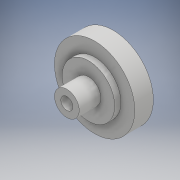
# Autodesk Inventor part: Arm - 608 bearing cap [Med]
Saved by Autodesk Inventor 2017 (Build 210142000, 142)
## iProperties
Created: 2016-08-10
Part Number: Arm - 608 bearing cap [Med]
Material: Generic
Document SubType Name: Modeling
Designer: Ali
Density: 1 g/cm^3
Appearance: Default
Author: Ali
Autodesk Inventor part; units mm, degrees
ref_plane "YZ Plane" through (0, 0, 0) normal (1, 0, 0) x (0, 1, 0)
ref_plane "XZ Plane" through (0, 0, 0) normal (0, 1, 0) x (-1, 0, 0)
ref_plane "XY Plane" through (0, 0, 0) normal (0, 0, 1) x (1, 0, 0)
sketch "Sketch1" plane through (0, 0, 0) normal (0, 1, 0) x (-1, 0, 0)
  circle A0 centre (0, 0) radius 8.5
  dimension "d0" = 17
  constraints: 1 centre point, 1 coincident
  measures "d0" diameter of A0
extrude "Extrusion1" add sketch "Sketch1" along normal blind 2
sketch "Sketch2" plane through (0, 2, 0) normal (0, 1, 0) x (1, 0, 0)
  circle A0 centre (0, 0) radius 13
  dimension "d3" = 26
  constraints: 1 centre point, 1 coincident
  measures "d3" diameter of A0
extrude "Extrusion2" add sketch "Sketch2" along normal blind 6
sketch "Sketch3" plane through (0, 0, 0) normal (0, -1, 0) x (1, 0, 0)
  circle A0 centre (0, 0) radius 4
  dimension "d6" = 8
  constraints: 1 centre point, 1 coincident
  measures "d6" diameter of A0
extrude "Extrusion3" add sketch "Sketch3" along normal blind 7
sketch "Sketch4" plane through (0, -7, 0) normal (0, -1, 0) x (1, 0, 0)
  point P0 (0, 0)
  point P1 (0, 0)
  constraints: 1 coincident
hole "Hole1" at (0, -7, 0) direction (0, 1, 0) diameter 3.9 depth 10 tip angle 118
sketch "Sketch6" plane through (0, 8, 0) normal (0, 1, 0) x (1, 0, 0)
  line L0 (5, 0) -> (-5, 0) construction
  line L1 (5, 0.9) -> (-5, 0.9)
  line L2 (-5, -0.9) -> (5, -0.9)
  arc A0 (5, -0.9) -> (5, 0.9) centre (5, 0) ccw
  arc A1 (-5, 0.9) -> (-5, -0.9) centre (-5, 0) ccw
  point P0 (0, 0)
  point P1 (0, 0)
  dimension "d24" = 1.8
  dimension "d25" = 10
  constraints: 8 end point, 4 point on circle, 4 tangent, 2 centre point, 1 coincident, 1 horizontal, 1 midpoint, 1 parallel
  measures "d24" diameter of A1
  measures "d25" distance of L0.end L0.start
extrude "Extrusion5" cut sketch "Sketch6" against normal blind 5
sketch "Sketch7" plane through (0, 8, 0) normal (0, 1, 0) x (1, 0, 0)
  line L0 (0.9699, -12.5028) -> (-0.9699, -12.5028)
  line L1 (-0.9699, -12.5028) -> (-0.9699, -13.4972)
  line L2 (-0.9699, -13.4972) -> (0.9699, -13.4972)
  line L3 (0.9699, -13.4972) -> (0.9699, -12.5028)
  circle A0 centre (0, 0) radius 13 projected
  line L4 (0.9699, -12.5028) -> (-0.9699, -13.4972) construction
  line L5 (-0.9699, -12.5028) -> (0.9699, -13.4972) construction
  circle A1 centre (0, 0) radius 13 projected
  line L6 (0, -13) -> (0, 0) construction
  constraints: 14 end point, 2 midpoint, 2 parallel, 1 horizontal, 1 perpendicular, 1 vertical, 1 vertical alignment, 1 other
body "Solid1"
